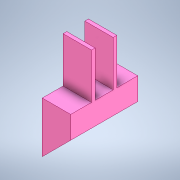
# Autodesk Inventor part: upperBracketForSquareBracket
Saved by Autodesk Inventor 2022.1 (Build 261234020, 234B)
## iProperties
Created: 2021-10-20
Part Number: upperBracketForSquareBracket
Material: PC/ABS Plastic
Document SubType Name: Modeling
Designer: robst
Density: 0.357273 g/cm^3
Appearance: Pink
Author: robst
Autodesk Inventor part; units mm, degrees
ref_plane "YZ Plane" through (0, 0, 0) normal (1, 0, 0) x (0, 1, 0)
ref_plane "XZ Plane" through (0, 0, 0) normal (0, 1, 0) x (-1, 0, 0)
ref_plane "XY Plane" through (0, 0, 0) normal (0, 0, 1) x (1, 0, 0)
sketch "Sketch55" plane through (0, 0, 0) normal (0, 0, 1) x (1, 0, 0)
  line L0 (0, 0) -> (0, -53.4597) construction
  line L1 (0, 0) -> (31.8198, 31.8198)
  line L2 (0, 0) -> (89.157, 0) construction
  line L3 (0, 0) -> (-31.8198, -31.8198)
  line L4 (31.8198, 31.8198) -> (-31.8198, 31.8198)
  line L5 (-31.8198, 31.8198) -> (-31.8198, -31.8198)
  dimension "d252" = 45
  constraints: 12 end point, 2 collinear, 2 horizontal, 2 vertical
  measures "d252" angle of L1 L2
extrude "Extrusion25" add sketch "Sketch55" along normal mid plane 150
sketch "Sketch56" plane through (-31.8198, 31.8198, 75) normal (0, 1, 0) x (1, 0, 0)
  line L0 (0, 150) -> (63.6396, 150) projected
  line L1 (63.6396, 0) -> (63.6396, 150) projected
  line L2 (0, 150) -> (0, 0) projected
  line L3 (63.6396, 0) -> (0, 0) projected
  line L4 (0, 150) -> (63.6396, 150)
  line L5 (63.6396, 150) -> (63.6396, 0)
  line L6 (63.6396, 0) -> (0, 0)
  line L7 (0, 0) -> (0, 150)
  point P0 (31.8198, 75)
  constraints: 8 end point, 2 parallel, 1 horizontal, 1 perpendicular
extrude "Extrusion26" add sketch "Sketch56" along normal blind 50
sketch "Sketch57" plane through (-31.8198, 81.8198, 75) normal (0, 1, 0) x (1, 0, 0)
  line L0 (63.6396, 150) -> (0, 150) projected
  line L1 (63.6396, 0) -> (63.6396, 150) projected
  line L2 (0, 0) -> (63.6396, 0) projected
  line L3 (0, 150) -> (0, 0) projected
  line L4 (0, 54.68) -> (63.6396, 54.68)
  line L5 (63.6396, 54.68) -> (63.6396, 95.32)
  line L6 (63.6396, 95.32) -> (0, 95.32)
  line L7 (0, 95.32) -> (0, 54.68)
  line L8 (0, 54.68) -> (63.6396, 95.32) construction
  line L9 (63.6396, 54.68) -> (0, 95.32) construction
  line L10 (0, 95.32) -> (63.6396, 95.32)
  line L11 (63.6396, 95.32) -> (63.6396, 103.42)
  line L12 (63.6396, 103.42) -> (0, 103.42)
  line L13 (0, 103.42) -> (0, 95.32)
  line L14 (0, 54.68) -> (63.6396, 54.68)
  line L15 (63.6396, 54.68) -> (63.6396, 46.58)
  line L16 (63.6396, 46.58) -> (0, 46.58)
  line L17 (0, 46.58) -> (0, 54.68)
  point P0 (31.8198, 75)
  point P1 (0, 46.58)
  point P2 (0, 103.42)
  point P3 (0, 95.32)
  dimension "d259" = 8.1
  dimension "d260" = 8.1
  dimension "d261" = 40.64
  constraints: 28 end point, 6 parallel, 3 perpendicular, 2 horizontal, 2 midpoint, 2 point on line
  measures "d259" distance between parallel lines of L12 L6
  measures "d260" distance between parallel lines of L16 L14
  measures "d261" distance of L6.end L4.start
extrude "Extrusion27" add sketch "Sketch57" along normal blind 101.6 contours L1 L6 L3 L12 | L1 L16 L3 L4
equation "\"d261\" = twoByFourWidth"
equation "\"wallThickness\" = 8"
equation "\"twoByFourWidth\" = 40.64"
equation "\"twoByFourDepth\" = 84.1375"
equation "\"azimuth\" = -15deg"
equation "\"elevation\" = 20deg"
equation "\"depthOfExtrusionForMatingToLowerHalf\" = 12.5"
equation "\"depthForWasherForMatingToCase\" = 14"
equation "\"topWallThickness\" = 8"
equation "\"widthOfCase\" = 149"
equation "\"sideWallThickness\" = 8"
equation "\"caseHeight\" = 125"
equation "\"bottomWallThickness\" = 8"
body "Solid4"
